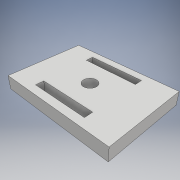
# Autodesk Inventor part: Female for pack
Saved by Autodesk Inventor 2018.1 (Build 221171000, 171)
## iProperties
Created: 2019-01-30
Part Number: Female for pack
Material: Типовые
Document SubType Name: Modeling
Designer: kostya
Density: 1 g/cm^3
Appearance: По умолчанию
Author: kostya
Autodesk Inventor part; units mm, degrees
ref_plane "YZ Plane" through (0, 0, 0) normal (1, 0, 0) x (0, 1, 0)
ref_plane "XZ Plane" through (0, 0, 0) normal (0, 1, 0) x (-1, 0, 0)
ref_plane "XY Plane" through (0, 0, 0) normal (0, 0, 1) x (1, 0, 0)
sketch "Эскиз1" plane through (0, 0, 0) normal (0, 0, 1) x (1, 0, 0)
  line L0 (-21, -15) -> (21, -15)
  line L1 (21, -15) -> (21, 15)
  line L2 (21, 15) -> (-21, 15)
  line L3 (-21, 15) -> (-21, -15)
  line L4 (-21, -15) -> (21, 15) construction
  line L5 (21, -15) -> (-21, 15) construction
  circle A0 centre (0, 0) radius 2.7
  line L6 (-10.7143, 15) -> (-10.7143, 12) construction
  line L7 (10.7143, 15) -> (10.7143, 13) construction
  line L8 (-10.7143, 12) -> (10, 12)
  line L9 (10, 12) -> (10, 9)
  line L10 (10, 9) -> (-10.7143, 9)
  line L11 (-10.7143, 9) -> (-10.7143, 12)
  line L12 (-21, 0) -> (21, 0) construction
  line L13 (-10.7143, -12) -> (10, -12)
  line L14 (10, -12) -> (10, -9)
  line L15 (-10.7143, -9) -> (-10.7143, -12)
  line L16 (10, -9) -> (-10.7143, -9)
  dimension "d0" = 42
  dimension "d1" = 30
  dimension "d2" = 5.4
  dimension "d3" = 3
  dimension "d4" = 2
  dimension "d5" = 3
  constraints: 34 end point, 4 midpoint, 4 parallel, 4 symmetric about line, 2 horizontal, 2 perpendicular, 2 point on line, 2 vertical, 1 centre point, 1 coincident
  measures "d0" distance of L2.end L1.end
  measures "d1" distance of L1.end L0.end
  measures "d2" diameter of A0
  measures "d3" distance of L6.start L6.end
  measures "d4" distance of L7.start L7.end
  measures "d5" distance of L8.end L9.end
extrude "Выдавливание1" add sketch "Эскиз1" along normal blind 5
